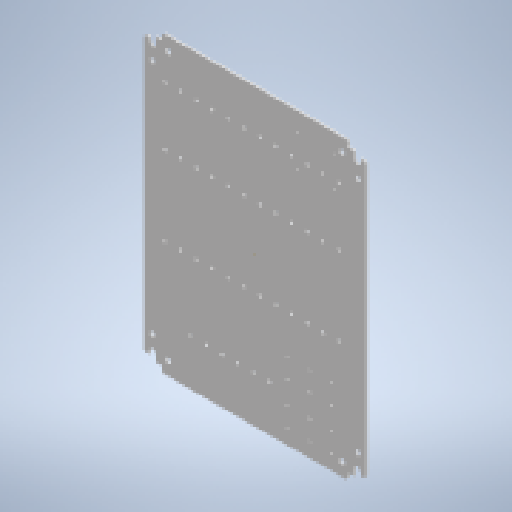
# Autodesk Inventor part: assembly-board
Saved by Autodesk Inventor 2023 (Build 270158030, 158C)
## iProperties
Created: 2024-03-20
Part Number: assembly-board
Material: Generic
Document SubType Name: Modeling
Designer: Imogen Heard
Density: 1 g/cm^3
Appearance: Default
Author: Imogen Heard
Autodesk Inventor part; units mm, degrees
ref_plane "YZ Plane" through (0, 0, 0) normal (1, 0, 0) x (0, 1, 0)
ref_plane "XZ Plane" through (0, 0, 0) normal (0, 1, 0) x (-1, 0, 0)
ref_plane "XY Plane" through (0, 0, 0) normal (0, 0, 1) x (1, 0, 0)
sketch "high voltage" plane through (0, 0, 0) normal (0, 0, 1) x (1, 0, 0)
  line L0 (-121.4929, -169.2156) -> (-167.7133, -169.2156)
  line L1 (-169.4454, -166.2156) -> (-146.3352, -126.1875)
  line L2 (-142.8711, -126.1875) -> (-119.7608, -166.2156)
  arc A0 (-142.8711, -126.1875) -> (-146.3352, -126.1875) centre (-144.6031, -127.1875) ccw
  arc A1 (-169.4454, -166.2156) -> (-167.7133, -169.2156) centre (-167.7133, -167.2156) ccw
  arc A2 (-121.4929, -169.2156) -> (-119.7608, -166.2156) centre (-121.4929, -167.2156) ccw
  line L3 (-145.4691, -126.6875) -> (-168.5793, -166.7156)
  arc A3 (-168.5793, -166.7156) -> (-167.7133, -168.2156) centre (-167.7133, -167.2156) ccw
  line L4 (-167.7133, -168.2156) -> (-121.4929, -168.2156)
  arc A4 (-121.4929, -168.2156) -> (-120.6269, -166.7156) centre (-121.4929, -167.2156) ccw
  line L5 (-120.6269, -166.7156) -> (-143.7371, -126.6875)
  arc A5 (-143.7371, -126.6875) -> (-145.4691, -126.6875) centre (-144.6031, -127.1875) ccw
  line L6 (-146.1782, -139.2847) -> (-142.8711, -139.2847)
  line L7 (-142.8711, -139.2847) -> (-147.4472, -150.1934)
  line L8 (-147.4472, -150.1934) -> (-140.7016, -147.4551)
  line L9 (-140.7016, -147.4551) -> (-144.0744, -160.167)
  line L10 (-144.0744, -160.167) -> (-142.8711, -160.167)
  line L11 (-142.8711, -160.167) -> (-145.822, -164.4859)
  line L12 (-145.822, -164.4859) -> (-147.4472, -160.0557)
  line L13 (-147.4472, -160.0557) -> (-146.1782, -160.0557)
  line L14 (-146.1782, -160.0557) -> (-143.8332, -151.8141)
  line L15 (-143.8332, -151.8141) -> (-150.3785, -154.471)
  line L16 (-150.3785, -154.471) -> (-146.1782, -139.2847)
  point P0 (-144.8622, -153.6861)
  point P1 (-144.6031, -153.8729)
  point P2 (-144.6031, -153.8729)
  point P3 (-118.0288, -169.2156)
  point P4 (-171.1774, -169.2156)
  point P5 (-144.6031, -123.1875)
  dimension "d142" = 2
  dimension "d146" = 1
  measures "d142" radius of A0
  measures "d146" distance between parallel lines of L3 L1
sketch "Sketch1" plane through (0, 0, 0) normal (0, 0, 1) x (1, 0, 0)
  line L0 (-175, 232.5) -> (175, 232.5)
  line L1 (175, 232.5) -> (175, -232.5)
  line L2 (175, -232.5) -> (-175, -232.5)
  line L3 (-175, -232.5) -> (-175, 232.5)
  point P0 (0, 0)
  dimension "d0" = 350
  dimension "d1" = 465
  dimension "d2" = 232.5
  dimension "d3" = 175
  constraints: 8 end point, 2 parallel, 1 horizontal, 1 perpendicular
  measures "d0" distance between parallel lines of L1 L3
  measures "d1" distance between parallel lines of L2 L0
  measures "d2" distance from line of point (0, 0) L0
  measures "d3" distance from line of point (0, 0) L1
extrude "Extrusion1" add sketch "Sketch1" along normal blind 3
sketch "Sketch3" plane through (0, 0, 3) normal (0, 0, 1) x (1, 0, 0)
  line L0 (-175, -232.5) -> (175, -232.5) projected
  line L1 (175, 232.5) -> (-175, 232.5) projected
  line L2 (175, -232.5) -> (175, 232.5) projected
  line L3 (-175, 232.5) -> (-175, -232.5) projected
  line L4 (-175, 232.5) -> (-146.5, 232.5)
  line L5 (-146.5, 232.5) -> (-146.5, 222.5)
  line L6 (-146.5, 222.5) -> (-175, 222.5)
  line L7 (-175, 222.5) -> (-175, 232.5)
  line L8 (-156, 216.5) -> (-175, 216.5)
  line L9 (-175, 216.5) -> (-175, 222.5)
  line L10 (-175, 222.5) -> (-156, 222.5)
  line L11 (-156, 222.5) -> (-156, 216.5)
  line L12 (-156, 216.5) -> (-167, 216.5)
  line L13 (-167, 216.5) -> (-167, 211.5)
  line L14 (-167, 211.5) -> (-156, 211.5)
  line L15 (-156, 211.5) -> (-156, 216.5)
  arc A0 (-167, 211.5) -> (-156, 211.5) centre (-161.5, 211.5) ccw
  line L16 (-146.5, 229.5) -> (-143.5, 232.5)
  line L17 (-175, 213.5) -> (-172, 216.5)
  circle A1 centre (-162, 187) radius 4.2
  circle A2 centre (-137.5, 211.5) radius 4.2
  point P0 (0, 0)
  dimension "d7" = 465
  dimension "d8" = 350
  dimension "d9" = 28.5
  dimension "d10" = 10
  dimension "d11" = 6
  dimension "d12" = 19
  dimension "d14" = 5
  dimension "d15" = 11
  dimension "d16" = 45
  dimension "d17" = 3
  dimension "d18" = 3
  dimension "d19" = 45
  dimension "d22" = 8.4
  dimension "d23" = 13
  dimension "d24" = 13.5
  dimension "d25" = 45.5
  dimension "d26" = 37.5
  dimension "d27" = 21
  constraints: 28 end point, 6 parallel, 3 centre point, 3 horizontal, 3 perpendicular, 3 point on line, 2 coincident, 2 point on circle, 1 equal radius, 1 horizontal alignment, 1 midpoint
  measures "d7" distance between parallel lines of L0 L1
  measures "d8" distance between parallel lines of L2 L3
  measures "d9" distance between parallel lines of L3 L5
  measures "d10" distance between parallel lines of L6 L1
  measures "d11" distance between parallel lines of L8 L6
  measures "d12" distance between parallel lines of L3 L11
  measures "d14" distance between parallel lines of L14 L12
  measures "d15" distance between parallel lines of L13 L15
  measures "d16" angle of L5 L16
  measures "d17" distance of L4.end L16.end
  measures "d18" distance from line of L3 L17.end
  measures "d19" angle of L8 L17
  measures "d22" diameter of A2
  measures "d23" distance from line of L3 A1.centre
  measures "d24" distance from line of L3 A0.centre
  measures "d25" distance from line of A1.centre L1
  measures "d26" distance from line of A2.centre L3
  measures "d27" distance from line of L1 A2.centre
extrude "Extrusion2" cut sketch "Sketch3" against normal through all contours L3 L8 L17 | L3 L6 L11 L8 | L16 L5 L1 | L3 L1 L5 L6 | L8 L15 L14 L13 | L14 A0 | A1 | A2
mirror "Mirror1" about plane through (0, 0, 0) normal (1, 0, 0) of "Extrusion2"
mirror "Mirror2" about plane through (0, 0, 0) normal (0, 1, 0) of "Extrusion2", "Mirror1"
sketch "Sketch4" plane through (0, 0, 3) normal (0, 0, 1) x (1, 0, 0)
  circle A0 centre (66.2112, 202.7338) radius 1.35 projected
  circle A1 centre (124.2112, 202.7338) radius 1.35 projected
  circle A2 centre (124.2112, 153.7338) radius 1.35 projected
  circle A3 centre (66.2112, 153.7338) radius 1.35 projected
  circle A4 centre (-142.425, 75.1905) radius 2.6
  arc A5 (113.375, 71.9905) -> (113.375, 78.3905) centre (113.375, 75.1905) ccw projected
  line L0 (113.375, 71.9905) -> (101.775, 71.9905) projected
  arc A6 (101.775, 78.3905) -> (101.775, 71.9905) centre (101.775, 75.1905) ccw projected
  line L1 (101.775, 78.3905) -> (113.375, 78.3905) projected
  arc A7 (-111.625, 71.9905) -> (-111.625, 78.3905) centre (-111.625, 75.1905) ccw projected
  line L2 (-111.625, 71.9905) -> (-123.225, 71.9905) projected
  arc A8 (-123.225, 78.3905) -> (-123.225, 71.9905) centre (-123.225, 75.1905) ccw projected
  line L3 (-123.225, 78.3905) -> (-111.625, 78.3905) projected
  arc A9 (13.375, 71.9905) -> (13.375, 78.3905) centre (13.375, 75.1905) ccw projected
  line L4 (13.375, 71.9905) -> (1.775, 71.9905) projected
  arc A10 (1.775, 78.3905) -> (1.775, 71.9905) centre (1.775, 75.1905) ccw projected
  line L5 (1.775, 78.3905) -> (13.375, 78.3905) projected
  arc A11 (-11.625, 71.9905) -> (-11.625, 78.3905) centre (-11.625, 75.1905) ccw projected
  line L6 (-11.625, 71.9905) -> (-23.225, 71.9905) projected
  arc A12 (-23.225, 78.3905) -> (-23.225, 71.9905) centre (-23.225, 75.1905) ccw projected
  line L7 (-23.225, 78.3905) -> (-11.625, 78.3905) projected
  arc A13 (-86.625, 71.9905) -> (-86.625, 78.3905) centre (-86.625, 75.1905) ccw projected
  line L8 (-86.625, 71.9905) -> (-98.225, 71.9905) projected
  arc A14 (-98.225, 78.3905) -> (-98.225, 71.9905) centre (-98.225, 75.1905) ccw projected
  line L9 (-98.225, 78.3905) -> (-86.625, 78.3905) projected
  arc A15 (88.375, 71.9905) -> (88.375, 78.3905) centre (88.375, 75.1905) ccw projected
  line L10 (88.375, 71.9905) -> (76.775, 71.9905) projected
  arc A16 (76.775, 78.3905) -> (76.775, 71.9905) centre (76.775, 75.1905) ccw projected
  line L11 (76.775, 78.3905) -> (88.375, 78.3905) projected
  arc A17 (138.375, 71.9905) -> (138.375, 78.3905) centre (138.375, 75.1905) ccw projected
  line L12 (138.375, 71.9905) -> (126.775, 71.9905) projected
  arc A18 (126.775, 78.3905) -> (126.775, 71.9905) centre (126.775, 75.1905) ccw projected
  line L13 (126.775, 78.3905) -> (138.375, 78.3905) projected
  arc A19 (-61.625, 71.9905) -> (-61.625, 78.3905) centre (-61.625, 75.1905) ccw projected
  line L14 (-61.625, 71.9905) -> (-73.225, 71.9905) projected
  arc A20 (-73.225, 78.3905) -> (-73.225, 71.9905) centre (-73.225, 75.1905) ccw projected
  line L15 (-73.225, 78.3905) -> (-61.625, 78.3905) projected
  arc A21 (38.375, 71.9905) -> (38.375, 78.3905) centre (38.375, 75.1905) ccw projected
  line L16 (38.375, 71.9905) -> (26.775, 71.9905) projected
  arc A22 (26.775, 78.3905) -> (26.775, 71.9905) centre (26.775, 75.1905) ccw projected
  line L17 (26.775, 78.3905) -> (38.375, 78.3905) projected
  arc A23 (-36.625, 71.9905) -> (-36.625, 78.3905) centre (-36.625, 75.1905) ccw projected
  line L18 (-36.625, 71.9905) -> (-48.225, 71.9905) projected
  arc A24 (-48.225, 78.3905) -> (-48.225, 71.9905) centre (-48.225, 75.1905) ccw projected
  line L19 (-48.225, 78.3905) -> (-36.625, 78.3905) projected
  line L20 (-148.225, 78.3905) -> (-136.625, 78.3905) projected
  arc A25 (-136.625, 71.9905) -> (-136.625, 78.3905) centre (-136.625, 75.1905) ccw projected
  line L21 (-136.625, 71.9905) -> (-148.225, 71.9905) projected
  arc A26 (-148.225, 78.3905) -> (-148.225, 71.9905) centre (-148.225, 75.1905) ccw projected
  arc A27 (63.375, 71.9905) -> (63.375, 78.3905) centre (63.375, 75.1905) ccw projected
  line L22 (63.375, 71.9905) -> (51.775, 71.9905) projected
  arc A28 (51.775, 78.3905) -> (51.775, 71.9905) centre (51.775, 75.1905) ccw projected
  line L23 (51.775, 78.3905) -> (63.375, 78.3905) projected
  line L24 (-155.025, 86.8905) -> (-155.025, 63.4905) projected
  line L25 (-155.025, 63.4905) -> (144.975, 63.4905) projected
  line L26 (144.975, 86.8905) -> (144.975, 63.4905) projected
  line L27 (-155.025, 86.8905) -> (144.975, 86.8905) projected
  circle A29 centre (-117.425, 75.1905) radius 2.6
  circle A30 centre (-92.425, 75.1905) radius 2.6
  circle A31 centre (-67.425, 75.1905) radius 2.6
  circle A32 centre (-42.425, 75.1905) radius 2.6
  circle A33 centre (-17.425, 75.1905) radius 2.6
  circle A34 centre (7.575, 75.1905) radius 2.6
  circle A35 centre (32.575, 75.1905) radius 2.6
  circle A36 centre (57.575, 75.1905) radius 2.6
  circle A37 centre (82.575, 75.1905) radius 2.6
  circle A38 centre (107.575, 75.1905) radius 2.6
  circle A39 centre (132.575, 75.1905) radius 2.6
  circle A40 centre (-142.425, -49.8095) radius 2.6
  circle A41 centre (-117.425, -49.8095) radius 2.6
  circle A42 centre (-92.425, -49.8095) radius 2.6
  circle A43 centre (-67.425, -49.8095) radius 2.6
  circle A44 centre (-42.425, -49.8095) radius 2.6
  circle A45 centre (-17.425, -49.8095) radius 2.6
  circle A46 centre (7.575, -49.8095) radius 2.6
  circle A47 centre (32.575, -49.8095) radius 2.6
  circle A48 centre (57.575, -49.8095) radius 2.6
  circle A49 centre (82.575, -49.8095) radius 2.6
  circle A50 centre (107.575, -49.8095) radius 2.6
  circle A51 centre (132.575, -49.8095) radius 2.6
  line L28 (24.975, -156.6095) -> (24.975, -148.1095) projected
  line L29 (-115.025, -148.1095) -> (24.975, -148.1095) projected
  line L30 (-115.025, -148.1095) -> (-115.025, -171.5095) projected
  line L31 (-115.025, -171.5095) -> (24.975, -171.5095) projected
  line L32 (24.975, -171.5095) -> (24.975, -163.0095) projected
  line L33 (24.975, -163.0095) -> (16.775, -163.0095) projected
  arc A52 (16.775, -156.6095) -> (16.775, -163.0095) centre (16.775, -159.8095) ccw projected
  line L34 (16.775, -156.6095) -> (24.975, -156.6095) projected
  arc A53 (-71.625, -163.0095) -> (-71.625, -156.6095) centre (-71.625, -159.8095) ccw projected
  line L35 (-71.625, -163.0095) -> (-83.225, -163.0095) projected
  arc A54 (-83.225, -156.6095) -> (-83.225, -163.0095) centre (-83.225, -159.8095) ccw projected
  line L36 (-83.225, -156.6095) -> (-71.625, -156.6095) projected
  arc A55 (-46.625, -163.0095) -> (-46.625, -156.6095) centre (-46.625, -159.8095) ccw projected
  line L37 (-46.625, -163.0095) -> (-58.225, -163.0095) projected
  arc A56 (-58.225, -156.6095) -> (-58.225, -163.0095) centre (-58.225, -159.8095) ccw projected
  line L38 (-58.225, -156.6095) -> (-46.625, -156.6095) projected
  arc A57 (-21.625, -163.0095) -> (-21.625, -156.6095) centre (-21.625, -159.8095) ccw projected
  line L39 (-21.625, -163.0095) -> (-33.225, -163.0095) projected
  arc A58 (-33.225, -156.6095) -> (-33.225, -163.0095) centre (-33.225, -159.8095) ccw projected
  line L40 (-33.225, -156.6095) -> (-21.625, -156.6095) projected
  arc A59 (3.375, -163.0095) -> (3.375, -156.6095) centre (3.375, -159.8095) ccw projected
  line L41 (3.375, -163.0095) -> (-8.225, -163.0095) projected
  arc A60 (-8.225, -156.6095) -> (-8.225, -163.0095) centre (-8.225, -159.8095) ccw projected
  line L42 (-8.225, -156.6095) -> (3.375, -156.6095) projected
  line L43 (-108.225, -156.6095) -> (-96.625, -156.6095) projected
  arc A61 (-96.625, -163.0095) -> (-96.625, -156.6095) centre (-96.625, -159.8095) ccw projected
  line L44 (-96.625, -163.0095) -> (-108.225, -163.0095) projected
  arc A62 (-108.225, -156.6095) -> (-108.225, -163.0095) centre (-108.225, -159.8095) ccw projected
  circle A63 centre (-102.425, -159.8095) radius 2.6
  circle A64 centre (-77.425, -159.8095) radius 2.6
  circle A65 centre (-52.425, -159.8095) radius 2.6
  circle A66 centre (-27.425, -159.8095) radius 2.6
  circle A67 centre (-2.425, -159.8095) radius 2.6
  circle A68 centre (22.575, -159.8095) radius 2.6
  arc A69 (49.282, -111.3926) -> (52.922, -111.3926) centre (51.102, -111.3926) ccw projected
  arc A70 (84.282, -111.3926) -> (87.922, -111.3926) centre (86.102, -111.3926) ccw projected
  arc A71 (119.282, -111.3926) -> (122.922, -111.3926) centre (121.102, -111.3926) ccw projected
  circle A72 centre (121.102, -142.2926) radius 1.82 projected
  circle A73 centre (86.102, -142.2926) radius 1.82 projected
  circle A74 centre (51.102, -142.2926) radius 1.82 projected
  circle A75 centre (51.102, -178.1926) radius 1.82 projected
  circle A76 centre (86.102, -178.1926) radius 1.82 projected
  circle A77 centre (121.102, -178.1926) radius 1.82 projected
  arc A78 (122.922, -209.0926) -> (119.282, -209.0926) centre (121.102, -209.0926) ccw projected
  arc A79 (87.922, -209.0926) -> (84.282, -209.0926) centre (86.102, -209.0926) ccw projected
  arc A80 (52.922, -209.0926) -> (49.282, -209.0926) centre (51.102, -209.0926) ccw projected
  circle A81 centre (51.102, -209.0926) radius 1.6
  circle A82 centre (86.102, -209.0926) radius 1.6
  circle A83 centre (121.102, -209.0926) radius 1.6
  circle A84 centre (51.102, -111.5926) radius 1.6
  circle A85 centre (86.102, -111.5926) radius 1.6
  circle A86 centre (121.102, -111.5926) radius 1.6
  circle A87 centre (-142.425, 167.1905) radius 2.6
  circle A88 centre (-117.425, 75.1905) radius 2.6
  circle A89 centre (-117.425, 167.1905) radius 2.6
  circle A90 centre (-92.425, 75.1905) radius 2.6
  circle A91 centre (-92.425, 167.1905) radius 2.6
  circle A92 centre (-67.425, 75.1905) radius 2.6
  circle A93 centre (-67.425, 167.1905) radius 2.6
  circle A94 centre (-42.425, 75.1905) radius 2.6
  circle A95 centre (-42.425, 167.1905) radius 2.6
  circle A96 centre (-17.425, 75.1905) radius 2.6
  circle A97 centre (-17.425, 167.1905) radius 2.6
  circle A98 centre (7.575, 75.1905) radius 2.6
  circle A99 centre (7.575, 167.1905) radius 2.6
  circle A100 centre (32.575, 75.1905) radius 2.6
  circle A101 centre (32.575, 167.1905) radius 2.6
  circle A102 centre (57.575, 75.1905) radius 2.6
  circle A103 centre (57.575, 167.1905) radius 2.6
  circle A104 centre (82.575, 75.1905) radius 2.6
  circle A105 centre (82.575, 167.1905) radius 2.6
  circle A106 centre (107.575, 75.1905) radius 2.6
  circle A107 centre (107.575, 167.1905) radius 2.6
  circle A108 centre (132.575, 75.1905) radius 2.6
  circle A109 centre (132.575, 167.1905) radius 2.6
  point P0 (0, 0)
  dimension "d28" = 5.2
  dimension "d29" = 5.8
  dimension "d30" = 5.8
  dimension "d31" = 25
  dimension "d34" = 25
  dimension "d37" = 125
  dimension "d40" = 5.2
  dimension "d41" = 5.8
  dimension "d44" = 25
  dimension "d49" = 3.2
  dimension "d52" = 35
  dimension "d55" = 97.5
  dimension "d60" = 92
  dimension "d63" = 25
  constraints: 59 centre point, 4 horizontal, 3 vertical, 2 horizontal alignment, 1 coincident, 112 other
  measures "d28" diameter of A4
  measures "d29" distance of A26.centre A4.centre
  measures "d30" distance of A25.centre A4.centre
  measures "d31" distance of A7.centre A25.centre
  measures "d34" distance of A4.centre A29.centre
  measures "d37" distance of A4.centre A40.centre
  measures "d40" diameter of A63
  measures "d41" distance of A62.centre A63.centre
  measures "d44" distance of A63.centre A64.centre
  measures "d49" diameter of A81
  measures "d52" distance of A81.centre A82.centre
  measures "d55" distance of A81.centre A84.centre
  measures "d60" distance of A4.centre A87.centre
  measures "d63" distance of A4.centre A88.centre
extrude "Extrusion3" cut sketch "Sketch4" against normal through all contours A0 | A1 | A2 | A3 | A4 | A29 | A30 | A31 | A32 | A33 | A34 | A35 | A36 | A37 | A38 | A39 | A40 | A41 | A42 | A43 | A44 | A45 | A46 | A47 | A48 | A49 | A50 | A51 | A63 | A64 | A65 | A66 | A67 | A68 | A72 | A73 | A74 | A75 | A76 | A77 | A81 | A82 | A83 | A84 | A85 | A86 | A87 | A89 | A91 | A93 | A95 | A97 | A99 | A101 | A103 | A105 | A107 | A109
sketch "Sketch5" plane through (0, 0, 3) normal (0, 0, 1) x (1, 0, 0)
  line L0 (-175, 213.5) -> (-175, -213.5) projected
  line L1 (-175, -87.5) -> (-160, -87.5)
  line L2 (-160, -87.5) -> (-160, -91.5)
  line L3 (-160, -91.5) -> (-175, -91.5)
  line L4 (-175, -91.5) -> (-175, -87.5)
  line L5 (-143.5, -232.5) -> (143.5, -232.5) projected
  line L6 (-150, -87.5) -> (-135, -87.5)
  line L7 (-135, -91.5) -> (-150, -91.5)
  line L8 (-135, -87.5) -> (-135, -91.5)
  line L9 (-150, -91.5) -> (-150, -87.5)
  line L10 (-125, -87.5) -> (-110, -87.5)
  line L11 (-110, -91.5) -> (-125, -91.5)
  line L12 (-110, -87.5) -> (-110, -91.5)
  line L13 (-125, -91.5) -> (-125, -87.5)
  line L14 (-100, -87.5) -> (-85, -87.5)
  line L15 (-85, -91.5) -> (-100, -91.5)
  line L16 (-85, -87.5) -> (-85, -91.5)
  line L17 (-100, -91.5) -> (-100, -87.5)
  line L18 (-75, -87.5) -> (-60, -87.5)
  line L19 (-60, -91.5) -> (-75, -91.5)
  line L20 (-60, -87.5) -> (-60, -91.5)
  line L21 (-75, -91.5) -> (-75, -87.5)
  line L22 (-50, -87.5) -> (-35, -87.5)
  line L23 (-35, -91.5) -> (-50, -91.5)
  line L24 (-35, -87.5) -> (-35, -91.5)
  line L25 (-50, -91.5) -> (-50, -87.5)
  line L26 (-25, -87.5) -> (-10, -87.5)
  line L27 (-10, -91.5) -> (-25, -91.5)
  line L28 (-10, -87.5) -> (-10, -91.5)
  line L29 (-25, -91.5) -> (-25, -87.5)
  line L30 (0, -87.5) -> (15, -87.5)
  line L31 (15, -91.5) -> (0, -91.5)
  line L32 (15, -87.5) -> (15, -91.5)
  line L33 (0, -91.5) -> (0, -87.5)
  line L34 (25, -87.5) -> (40, -87.5)
  line L35 (40, -91.5) -> (25, -91.5)
  line L36 (40, -87.5) -> (40, -91.5)
  line L37 (25, -91.5) -> (25, -87.5)
  line L38 (50, -87.5) -> (65, -87.5)
  line L39 (65, -91.5) -> (50, -91.5)
  line L40 (65, -87.5) -> (65, -91.5)
  line L41 (50, -91.5) -> (50, -87.5)
  line L42 (75, -91.5) -> (75, -87.5)
  line L43 (90, -91.5) -> (75, -91.5)
  line L44 (90, -87.5) -> (90, -91.5)
  line L45 (75, -87.5) -> (90, -87.5)
  line L46 (100, -91.5) -> (100, -87.5)
  line L47 (115, -91.5) -> (100, -91.5)
  line L48 (115, -87.5) -> (115, -91.5)
  line L49 (100, -87.5) -> (115, -87.5)
  line L50 (125, -91.5) -> (125, -87.5)
  line L51 (140, -91.5) -> (125, -91.5)
  line L52 (140, -87.5) -> (140, -91.5)
  line L53 (125, -87.5) -> (140, -87.5)
  line L54 (150, -91.5) -> (150, -87.5)
  line L55 (165, -91.5) -> (150, -91.5)
  line L56 (165, -87.5) -> (165, -91.5)
  line L57 (150, -87.5) -> (165, -87.5)
  line L58 (-84.5169, -96.4994) -> (24.8633, -96.4994) construction
  line L59 (24.8633, -96.4994) -> (24.8633, -107.8996) construction
  line L60 (24.8633, -107.8996) -> (-84.5169, -107.8996) construction
  line L61 (-84.5169, -107.8996) -> (-84.5169, -96.4994) construction
  line L62 (-67.4562, -118.0258) -> (-47.9562, -118.0258)
  line L63 (-47.9562, -118.0258) -> (-47.9562, -203.2928)
  line L64 (-47.9562, -203.2928) -> (-67.4562, -203.2928)
  line L65 (-67.4562, -203.2928) -> (-67.4562, -118.0258)
  line L66 (-48.9562, -202.2928) -> (-48.9562, -119.0258)
  line L67 (-48.9562, -119.0258) -> (-66.4562, -119.0258)
  line L68 (-66.4562, -119.0258) -> (-66.4562, -202.2928)
  line L69 (-66.4562, -202.2928) -> (-48.9562, -202.2928)
  line L70 (-29.4562, -119.0258) -> (-46.9562, -119.0258)
  line L71 (-47.9562, -118.0258) -> (-28.4562, -118.0258)
  line L72 (-29.4562, -202.2928) -> (-29.4562, -119.0258)
  line L73 (-46.9562, -119.0258) -> (-46.9562, -202.2928)
  line L74 (-28.4562, -118.0258) -> (-28.4562, -203.2928)
  line L75 (-46.9562, -202.2928) -> (-29.4562, -202.2928)
  line L76 (-28.4562, -203.2928) -> (-47.9562, -203.2928)
  line L77 (-47.9562, -203.2928) -> (-47.9562, -118.0258)
  line L78 (-9.9562, -119.0258) -> (-27.4562, -119.0258)
  line L79 (-28.4562, -118.0258) -> (-8.9562, -118.0258)
  line L80 (-9.9562, -202.2928) -> (-9.9562, -119.0258)
  line L81 (-27.4562, -119.0258) -> (-27.4562, -202.2928)
  line L82 (-8.9562, -118.0258) -> (-8.9562, -203.2928)
  line L83 (-27.4562, -202.2928) -> (-9.9562, -202.2928)
  line L84 (-8.9562, -203.2928) -> (-28.4562, -203.2928)
  line L85 (-28.4562, -203.2928) -> (-28.4562, -118.0258)
  line L86 (9.5438, -119.0258) -> (-7.9562, -119.0258)
  line L87 (-8.9562, -118.0258) -> (10.5438, -118.0258)
  line L88 (9.5438, -202.2928) -> (9.5438, -119.0258)
  line L89 (-7.9562, -119.0258) -> (-7.9562, -202.2928)
  line L90 (10.5438, -118.0258) -> (10.5438, -203.2928)
  line L91 (-7.9562, -202.2928) -> (9.5438, -202.2928)
  line L92 (10.5438, -203.2928) -> (-8.9562, -203.2928)
  line L93 (-8.9562, -203.2928) -> (-8.9562, -118.0258)
  line L94 (29.0438, -119.0258) -> (11.5438, -119.0258)
  line L95 (10.5438, -118.0258) -> (30.0438, -118.0258)
  line L96 (29.0438, -202.2928) -> (29.0438, -119.0258)
  line L97 (11.5438, -119.0258) -> (11.5438, -202.2928)
  line L98 (30.0438, -118.0258) -> (30.0438, -203.2928)
  line L99 (11.5438, -202.2928) -> (29.0438, -202.2928)
  line L100 (30.0438, -203.2928) -> (10.5438, -203.2928)
  line L101 (10.5438, -203.2928) -> (10.5438, -118.0258)
  line L102 (-59.7232, -120.1793) -> (-51.7369, -120.1793) construction
  line L103 (-51.7369, -120.1793) -> (-51.7369, -126.2793) construction
  line L104 (-51.7369, -126.2793) -> (-59.7232, -126.2793) construction
  line L105 (-59.7232, -126.2793) -> (-59.7232, -120.1793) construction
  line L106 (-42.5354, -120.1793) -> (-31.6524, -120.1793) construction
  line L107 (-31.6524, -120.1793) -> (-31.6524, -126.2793) construction
  line L108 (-31.6524, -126.2793) -> (-42.5354, -126.2793) construction
  line L109 (-42.5354, -126.2793) -> (-42.5354, -120.1793) construction
  line L110 (-3.0255, -126.2793) -> (-3.0255, -120.1793) construction
  line L111 (-3.0255, -120.1793) -> (5.8128, -120.1793) construction
  line L112 (5.8128, -120.1793) -> (5.8128, -126.2793) construction
  line L113 (5.8128, -126.2793) -> (-3.0255, -126.2793) construction
  line L114 (-22.6436, -126.2793) -> (-22.6436, -120.1793) construction
  line L115 (-22.6436, -120.1793) -> (-13.8054, -120.1793) construction
  line L116 (-13.8054, -120.1793) -> (-13.8054, -126.2793) construction
  line L117 (-13.8054, -126.2793) -> (-22.6436, -126.2793) construction
  line L118 (16.0367, -126.2793) -> (16.0367, -120.1793) construction
  line L119 (16.0367, -120.1793) -> (24.8749, -120.1793) construction
  line L120 (24.8749, -120.1793) -> (24.8749, -126.2793) construction
  line L121 (24.8749, -126.2793) -> (16.0367, -126.2793) construction
  line L122 (-110, 10.5365) -> (-60, 10.5365)
  line L123 (-60, 10.5365) -> (-60, -84.0099)
  line L124 (-60, -84.0099) -> (-110, -84.0099)
  line L125 (-110, -84.0099) -> (-110, 10.5365)
  line L126 (-60, 10.5365) -> (2, 10.5365)
  line L127 (2, 10.5365) -> (2, -84.0099)
  line L128 (2, -84.0099) -> (-60, -84.0099)
  line L129 (-60, -84.0099) -> (-60, 10.5365)
  line L130 (2, 10.5365) -> (22, 10.5365)
  line L131 (22, 10.5365) -> (22, -84.0099)
  line L132 (22, -84.0099) -> (2, -84.0099)
  line L133 (2, -84.0099) -> (2, 10.5365)
  line L134 (-61, 9.5365) -> (-109, 9.5365)
  line L135 (-109, 9.5365) -> (-109, -83.0099)
  line L136 (-109, -83.0099) -> (-61, -83.0099)
  line L137 (-61, -83.0099) -> (-61, 9.5365)
  line L138 (3, 9.5365) -> (21, 9.5365)
  line L139 (21, 9.5365) -> (21, -83.0099)
  line L140 (21, -83.0099) -> (3, -83.0099)
  line L141 (3, -83.0099) -> (3, 9.5365)
  line L142 (-59, 9.5365) -> (1, 9.5365)
  line L143 (1, 9.5365) -> (1, -83.0099)
  line L144 (1, -83.0099) -> (-59, -83.0099)
  line L145 (-59, -83.0099) -> (-59, 9.5365)
  line L146 (-91.3061, 0.557) -> (-91.3061, 6.657) construction
  line L147 (-91.3061, 6.657) -> (-75.4153, 6.657) construction
  line L148 (-75.4153, 6.657) -> (-75.4153, 0.557) construction
  line L149 (-75.4153, 0.557) -> (-91.3061, 0.557) construction
  line L150 (-37.021, 0.7734) -> (-37.021, 6.8734) construction
  line L151 (-37.021, 6.8734) -> (-21.1303, 6.8734) construction
  line L152 (-21.1303, 6.8734) -> (-21.1303, 0.7734) construction
  line L153 (-21.1303, 0.7734) -> (-37.021, 0.7734) construction
  line L154 (3.7464, 2.4981) -> (3.7464, 8.5981) construction
  line L155 (3.7464, 8.5981) -> (19.6371, 8.5981) construction
  line L156 (19.6371, 8.5981) -> (19.6371, 2.4981) construction
  line L157 (19.6371, 2.4981) -> (3.7464, 2.4981) construction
  point P0 (0, 0)
  dimension "d68" = 4
  dimension "d69" = 15
  dimension "d70" = 145
  dimension "d73" = 25
  dimension "d83" = 25
  dimension "d148" = 19.5
  dimension "d150" = 1
  dimension "d157" = 19.5
  dimension "d176" = 50
  dimension "d177" = 62
  dimension "d178" = 20
  dimension "d179" = 1
  dimension "d180" = 1
  dimension "d181" = 1
  dimension "d182" = 1
  dimension "d183" = 1
  dimension "d184" = 1
  constraints: 240 end point, 18 parallel, 9 horizontal, 9 perpendicular, 4 horizontal alignment, 1 point on line, 195 other
  measures "d68" distance between parallel lines of L3 L1
  measures "d69" distance between parallel lines of L0 L2
  measures "d70" distance between parallel lines of L5 L1
  measures "d73" distance of L1.start L6.start
  measures "d83" distance of L38.start L42.end
  measures "d148" distance between parallel lines of L63 L65
  measures "d150" distance between parallel lines of L63 L66
  measures "d157" distance of L62.end L71.end
  measures "d176" distance between parallel lines of L123 L125
  measures "d177" distance between parallel lines of L127 L123
  measures "d178" distance between parallel lines of L131 L133
  measures "d179" distance between parallel lines of L122 L134
  measures "d180" distance between parallel lines of L126 L142
  measures "d181" distance between parallel lines of L123 L145
  measures "d182" distance between parallel lines of L127 L143
  measures "d183" distance between parallel lines of L128 L144
  measures "d184" distance between parallel lines of L130 L138
equation "\"d2\" = 0.5 * d1"
equation "\"d3\" = 0.5 * d0"
body "Solid1"
